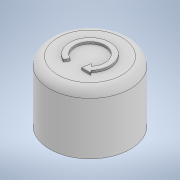
# Autodesk Inventor part: Device Rotation Button
Saved by Autodesk Inventor 2021 (Build 250183000, 183)
## iProperties
Created: 2021-03-24
Part Number: Device Rotation Button
Material: Generic
Document SubType Name: Modeling
Designer: eng1-127
Density: 1 g/cm^3
Appearance: Default
Author: eng1-127
Autodesk Inventor part; units mm, degrees
ref_plane "YZ Plane" through (0, 0, 0) normal (1, 0, 0) x (0, 1, 0)
ref_plane "XZ Plane" through (0, 0, 0) normal (0, 1, 0) x (-1, 0, 0)
ref_plane "XY Plane" through (0, 0, 0) normal (0, 0, 1) x (1, 0, 0)
sketch "Sketch1" plane through (0, 0, 0) normal (0, 1, 0) x (-1, 0, 0)
  circle A0 centre (0, 0) radius 10
  dimension "d0" = 20
  constraints: 1 centre point, 1 coincident
  measures "d0" diameter of A0
extrude "Extrusion1" add sketch "Sketch1" along normal blind 15
sketch "Sketch2" plane through (0, 0, 0) normal (0, -1, 0) x (1, 0, 0)
  circle A0 centre (0, 0) radius 7.5
  dimension "d3" = 15
  constraints: 1 centre point, 1 coincident
  measures "d3" diameter of A0
extrude "Extrusion2" cut sketch "Sketch2" against normal blind 5
fillet "Fillet1" radius 2 1 edges at (10, 15, 0)
sketch "Sketch4" plane through (0, 15, 0) normal (0, 1, 0) x (1, 0, 0)
  arc A0 (2.7981, -2.4967) -> (-1.483, -3.4443) centre (0, 0) ccw
  arc A1 (3.6613, -3.4051) -> (-2.1245, -4.5262) centre (0, 0) ccw
  line L0 (-2.1245, -4.5262) -> (-1.483, -3.4443)
  line L1 (1.8934, -3.9852) -> (2.2247, -1.8934)
  line L2 (4.2127, -3.9852) -> (1.8934, -3.9852)
  line L3 (2.2247, -1.8934) -> (2.7981, -2.4967)
  line L4 (3.6613, -3.4051) -> (4.2127, -3.9852)
  dimension "d12" = 7.5
  dimension "d13" = 10
  constraints: 10 end point, 4 point on circle, 2 centre point, 2 coincident, 1 horizontal
  measures "d12" diameter of A0
  measures "d13" diameter of A1
extrude "Extrusion4" add sketch "Sketch4" along normal blind 0.5
body "Solid1"
